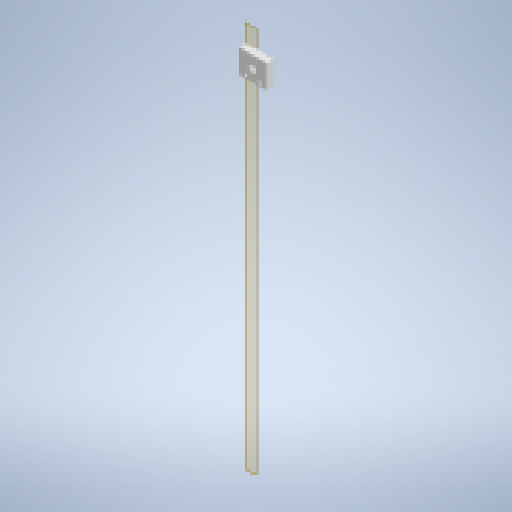
# Autodesk Inventor part: ender
Saved by Autodesk Inventor 2024 (Build 280153000, 153)
## iProperties
Created: 2026-03-01
Part Number: ender
Material: Generic
Document SubType Name: Modeling
Designer: SEMEN
Density: 1 g/cm^3
Appearance: Default
Author: SEMEN
Autodesk Inventor part; units mm, degrees
ref_plane "YZ Plane" through (0, 0, 0) normal (1, 0, 0) x (0, 1, 0)
ref_plane "XZ Plane" through (0, 0, 0) normal (0, 1, 0) x (-1, 0, 0)
ref_plane "XY Plane" through (0, 0, 0) normal (0, 0, 1) x (1, 0, 0)
ref_plane "Work Plane1" through (0, 0, 0) normal (0, 0, 1) x (1, 0, 0)
sketch "Sketch1" plane through (0, 0, 0) normal (0, 0, 1) x (1, 0, 0)
  line L0 (0, 750) -> (7, 750) projected
  line L1 (7, 750) -> (7, 1000) projected
  line L2 (0, 1000) -> (7, 1000) projected
  line L3 (0, 750) -> (0, 1000) projected
  line L4 (13, 750) -> (20, 750) projected
  line L5 (20, 750) -> (20, 1000) projected
  line L6 (13, 1000) -> (20, 1000) projected
  line L7 (13, 750) -> (13, 1000) projected
  line L8 (0, 1000) -> (20, 1000)
  line L9 (20, 1000) -> (20, 983)
  line L10 (20, 983) -> (0, 983)
  line L11 (0, 983) -> (0, 1000)
  line L12 (10, 1000) -> (10, 983) construction
  circle A0 centre (10, 991.5) radius 4.5 construction
  line L13 (0, 985.5) -> (20, 985.5) construction
  point P0 (0, 0)
  point P1 (5.25, 985.5)
  point P2 (14.75, 985.5)
  point P3 (0, 983)
  dimension "d0" = 9
  dimension "d3" = 9.5
  dimension "d4" = 2.5
  dimension "d5" = 17
  constraints: 12 end point, 5 point on line, 3 midpoint, 2 parallel, 2 perpendicular, 1 centre point, 1 coincident, 1 horizontal, 1 symmetric about line
  measures "d0" diameter of A0
  measures "d3" distance of point (14.75, 985.5) point (5.25, 985.5)
  measures "d4" distance between parallel lines of L10 L13
  measures "d5" distance between parallel lines of L6 L10
extrude "Extrusion1" add sketch "Sketch1" along normal blind 5 contours L3 L2 L1 L10 | L1 L8 L7 L10 | L7 L6 L5 L10
hole "Hole1" at (5.25, 985.5, 0) at (14.75, 985.5, 0) direction (0, 0, 1) diameter 2.4 end through all clearance for "Hex Head Bolt / Nut GOST 12876-67" size "M2" standard "GOST"
hole "Hole2" at (10, 991.5, 0) direction (0, 0, 1) diameter 4.5 end through all clearance for "Hex Head Bolt / Nut GOST 12876-67" size "M4" standard "GOST"
sketch "Sketch2" plane through (0, 0, 0) normal (0, 0, -1) x (-1, 0, 0)
  circle A0 centre (-14.75, 985.5) radius 1.2 projected
  circle A1 centre (-5.25, 985.5) radius 1.2 projected
  line L0 (-12.75, 984.3453) -> (-14.75, 983.1906)
  line L1 (-14.75, 983.1906) -> (-16.75, 984.3453)
  line L2 (-16.75, 984.3453) -> (-16.75, 986.6547)
  line L3 (-16.75, 986.6547) -> (-14.75, 987.8094)
  line L4 (-14.75, 987.8094) -> (-12.75, 986.6547)
  line L5 (-12.75, 986.6547) -> (-12.75, 984.3453)
  line L6 (-7.25, 984.3453) -> (-7.25, 986.6547)
  line L7 (-7.25, 986.6547) -> (-5.25, 987.8094)
  line L8 (-5.25, 987.8094) -> (-3.25, 986.6547)
  line L9 (-3.25, 986.6547) -> (-3.25, 984.3453)
  line L10 (-3.25, 984.3453) -> (-5.25, 983.1906)
  line L11 (-5.25, 983.1906) -> (-7.25, 984.3453)
  line L12 (-20, 983) -> (-20, 1000) projected
  point P0 (0, 0)
  dimension "d22" = 4
  constraints: 24 end point, 3 parallel, 2 coincident, 26 other
  measures "d22" distance between parallel lines of L5 L2
extrude "Extrusion2" cut sketch "Sketch2" against normal blind 2
body "Solid1"
